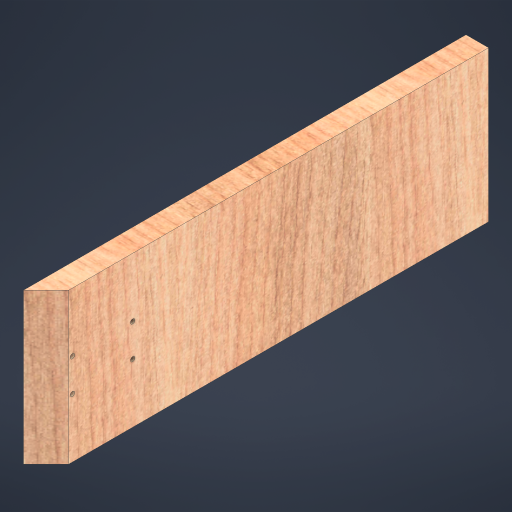
# Autodesk Inventor part: BUMP_002_Wood2
Saved by Autodesk Inventor 2024.2 (Build 282272000, 272)
## iProperties
Created: 2024-08-06
Part Number: BUMP_002_Wood2
Material: Wood (Birch)
Document SubType Name: Modeling
Designer: Bryan
Density: 0.55 g/cm^3
Appearance: Birch - Natural Polished
Author: Bryan
Autodesk Inventor part; units mm, degrees
ref_plane "YZ Plane" through (0, 0, 0) normal (1, 0, 0) x (0, 1, 0)
ref_plane "XZ Plane" through (0, 0, 0) normal (0, 1, 0) x (-1, 0, 0)
ref_plane "XY Plane" through (0, 0, 0) normal (0, 0, 1) x (1, 0, 0)
sketch "Sketch2" plane through (0, 0, 0) normal (0, 1, 0) x (-1, 0, 0)
  line L0 (0, 0) -> (0, -711.2)
  line L1 (19.05, 19.05) -> (19.05, -730.25)
  line L2 (19.05, -730.25) -> (0, -711.2)
  line L3 (19.05, 19.05) -> (0, 0)
  point P0 (19.05, -355.6)
  point P1 (0, -355.6)
  dimension "d2" = 711.2
  dimension "d3" = 749.3
  dimension "d4" = 19.05
  constraints: 8 end point, 2 midpoint, 2 vertical, 1 horizontal alignment
  measures "d2" distance of L0.start L0.end
  measures "d3" distance of L1.start L1.end
  measures "d4" distance between parallel lines of L0 L1
extrude "Extrusion1" add sketch "Sketch2" along normal blind 127
sketch "Sketch3" plane through (0, 0, 0) normal (1, 0, 0) x (0, 0, -1)
  line L0 (0, 0) -> (711.2, 0) construction
  line L1 (711.2, 0) -> (711.2, 127) construction
  line L2 (0, 127) -> (711.2, 127) construction
  line L3 (0, 0) -> (0, 127) construction
  line L4 (0, 77.2583) -> (3.175, 77.2583) construction
  circle A0 centre (3.175, 77.2583) radius 1.905
  circle A1 centre (53.975, 77.2583) radius 1.905
  circle A2 centre (104.775, 77.2583) radius 1.905 construction
  circle A3 centre (3.175, 49.7417) radius 1.905
  circle A4 centre (53.975, 49.7417) radius 1.905
  circle A5 centre (104.775, 49.7417) radius 1.905 construction
  line L5 (355.6, 127) -> (355.6, 0) construction
  circle A6 centre (708.025, 77.2583) radius 1.905
  circle A7 centre (657.225, 77.2583) radius 1.905
  circle A8 centre (606.425, 77.2583) radius 1.905 construction
  circle A9 centre (708.025, 49.7417) radius 1.905
  circle A10 centre (657.225, 49.7417) radius 1.905
  circle A11 centre (606.425, 49.7417) radius 1.905 construction
  line L6 (3.175, 77.2583) -> (3.175, 49.7417) construction
  line L7 (-19.05, 0) -> (-19.05, 127) projected
  point P0 (3.175, 63.5)
  dimension "d9" = 3.81
  dimension "d12" = 50.8
  dimension "d15" = 27.5167
  dimension "d23" = 63.5
  dimension "d24" = 22.225
  constraints: 12 centre point, 7 symmetric about line, 6 end point, 3 midpoint, 2 coincident, 2 horizontal, 2 vertical, 1 point on line, 16 other
  measures "d9" diameter of A0
  measures "d12" distance of L6.start A1.centre
  measures "d15" distance of L6.start L6.end
  measures "d23" distance from line of L2 point (3.175, 63.5)
  measures "d24" distance between parallel lines of L7 L6
extrude "Extrusion2" cut sketch "Sketch3" against normal blind 127
sketch "Sketch4" plane through (0, 127, 0) normal (0, 1, 0) x (1, 0, 0)
  line L0 (-19.05, 730.25) -> (-19.05, -19.05) projected
  line L1 (-19.05, 355.6) -> (0, 355.6)
  line L2 (0, 0) -> (0, 711.2) projected
  line L3 (0, 0) -> (0, 711.2) projected
  line L4 (0, 711.2) -> (-19.05, 730.25) projected
  line L5 (-19.05, 730.25) -> (-19.05, -19.05) projected
  line L6 (-19.05, -19.05) -> (0, 0) projected
  line L7 (-19.05, 354.0125) -> (0, 354.0125)
  dimension "d22" = 1.5875
  constraints: 4 end point, 2 midpoint, 2 point on line, 1 horizontal
  measures "d22" distance between parallel lines of L7 L1
extrude "Extrusion3" cut sketch "Sketch4" against normal blind 127 contours L4 L2 L1 L0 | L1 L2 L7 L0
body "Solid1"
